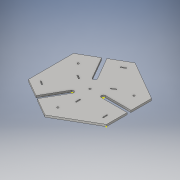
# Autodesk Inventor part: servo mount
Saved by Autodesk Inventor 2016 (Build 200138000, 138)
## iProperties
Created: 2016-04-10
Part Number: servo mount
Material: Generic
Document SubType Name: Modeling
Designer: Sam
Density: 1 g/cm^3
Appearance: Default
Author: Sam
Autodesk Inventor part; units mm, degrees
ref_plane "YZ Plane" through (0, 0, 0) normal (1, 0, 0) x (0, 1, 0)
ref_plane "XZ Plane" through (0, 0, 0) normal (0, 1, 0) x (-1, 0, 0)
ref_plane "XY Plane" through (0, 0, 0) normal (0, 0, 1) x (1, 0, 0)
sketch "Sketch1" plane through (0, 0, 0) normal (0, 1, 0) x (-1, 0, 0)
  point P0 (0, 0)
sketch "Sketch2" plane through (0, 0, 0) normal (0, 1, 0) x (-1, 0, 0)
  line L0 (0, 0) -> (0, -70)
  line L1 (0, -70) -> (54.3409, -70) construction
  line L2 (0, -70) -> (60.6218, -105)
  line L3 (0, -70) -> (70, -70) construction
  line L4 (60.6218, -105) -> (121.2436, -70)
  line L5 (121.2436, -70) -> (121.2436, 0)
  line L6 (121.2436, 0) -> (60.6218, 35)
  line L7 (60.6218, 35) -> (0, 0)
  dimension "d0" = 70
  dimension "d2" = 70
  dimension "d3" = 30
  dimension "d4" = 70
  dimension "d5" = 120
  dimension "d6" = 70
  dimension "d7" = 120
  constraints: 16 end point, 2 horizontal, 2 parallel, 2 vertical, 1 equal length
  measures "d0" distance of L0.start L0.end
  measures "d2" distance of L0.end L2.end
  measures "d3" angle of L2 L3
  measures "d4" distance of L2.end L4.end
  measures "d5" angle of L4 L2
  measures "d6" distance of L5.end L6.end
  measures "d7" angle of L6 L5
extrude "Extrusion1" add sketch "Sketch2" along normal blind 3
sketch "Sketch3" plane through (0, 3, 0) normal (0, 1, 0) x (1, 0, 0)
  line L0 (0, 0) -> (0, 70) projected
  line L1 (-121.2436, 0) -> (-60.6218, -35) projected
  line L2 (-90.9327, -17.5) -> (-50.9327, -17.5) construction
  line L3 (-60.6218, 105) -> (-121.2436, 70) projected
  line L4 (-90.9327, 87.5) -> (-50.9327, 87.5) construction
  line L5 (-70.9327, 17.141) -> (-90.9327, -17.5) construction
  line L6 (-73.5307, 18.641) -> (-93.5307, -16)
  line L7 (-88.3346, -19) -> (-68.3346, 15.641)
  arc A0 (-68.3346, 15.641) -> (-73.5307, 18.641) centre (-70.9327, 17.141) ccw
  arc A1 (-93.5307, -16) -> (-88.3346, -19) centre (-90.9327, -17.5) ccw
  line L8 (-70.9327, 52.859) -> (-90.9327, 87.5) construction
  line L9 (-68.3346, 54.359) -> (-88.3346, 89)
  line L10 (-93.5307, 86) -> (-73.5307, 51.359)
  arc A2 (-73.5307, 51.359) -> (-68.3346, 54.359) centre (-70.9327, 52.859) ccw
  arc A3 (-88.3346, 89) -> (-93.5307, 86) centre (-90.9327, 87.5) ccw
  line L11 (-40, 35) -> (0, 35) construction
  line L12 (-40, 32) -> (0, 32)
  line L13 (0, 38) -> (-40, 38)
  arc A4 (-40, 38) -> (-40, 32) centre (-40, 35) ccw
  arc A5 (0, 32) -> (0, 38) centre (0, 35) ccw
  point P0 (-80.9327, -0.1795)
  point P1 (-80.9327, 70.1795)
  point P2 (-20, 35)
  dimension "d10" = 40
  dimension "d11" = 40
  dimension "d13" = 40
  dimension "d15" = 6
  dimension "d16" = 6
  dimension "d17" = 6
  constraints: 28 end point, 12 point on circle, 12 tangent, 6 centre point, 6 midpoint, 3 parallel, 2 horizontal, 1 perpendicular
  measures "d10" distance of L11.end L11.start
  measures "d11" distance of L2.start L5.start
  measures "d13" distance of L4.start L8.start
  measures "d15" diameter of A1
  measures "d16" diameter of A3
  measures "d17" diameter of A5
extrude "Extrusion3" cut sketch "Sketch3" against normal blind 3
sketch "Sketch4" plane through (0, 3, 0) normal (0, 1, 0) x (1, 0, 0)
  line L0 (-54, 7) -> (-54, 13) construction
  line L1 (-53.25, 7) -> (-53.25, 13)
  line L2 (-54.75, 13) -> (-54.75, 7)
  arc A0 (-54.75, 7) -> (-53.25, 7) centre (-54, 7) ccw
  arc A1 (-53.25, 13) -> (-54.75, 13) centre (-54, 13) ccw
  line L3 (-54, 10) -> (-48, 10) construction
  line L4 (-12, 7) -> (-12, 13) construction
  line L5 (-11.25, 7) -> (-11.25, 13)
  line L6 (-12.75, 13) -> (-12.75, 7)
  arc A2 (-12.75, 7) -> (-11.25, 7) centre (-12, 7) ccw
  arc A3 (-11.25, 13) -> (-12.75, 13) centre (-12, 13) ccw
  line L7 (-12, 10) -> (-6, 10) construction
  arc A4 (-40, 38) -> (-40, 32) centre (-40, 35) ccw projected
  line L8 (-121.2436, 70) -> (-121.2436, 0) projected
  arc A5 (-73.5307, 51.359) -> (-68.3346, 54.359) centre (-70.9327, 52.859) ccw projected
  line L9 (-60.6218, -35) -> (0, 0) projected
  line L10 (-42.282, 53.2346) -> (-45.282, 58.4308) construction
  line L11 (-39.684, 54.7346) -> (-44.8801, 51.7346) construction
  arc A6 (-45.2551, 52.3841) -> (-44.5051, 51.0851) centre (-44.8801, 51.7346) ccw
  line L12 (-44.5051, 51.0851) -> (-39.309, 54.0851)
  arc A7 (-39.309, 54.0851) -> (-40.059, 55.3841) centre (-39.684, 54.7346) ccw
  line L13 (-40.059, 55.3841) -> (-45.2551, 52.3841)
  line L14 (-65.5051, 87.4582) -> (-60.309, 90.4582)
  arc A8 (-60.309, 90.4582) -> (-61.059, 91.7572) centre (-60.684, 91.1077) ccw
  arc A9 (-66.2551, 88.7572) -> (-65.5051, 87.4582) centre (-65.8801, 88.1077) ccw
  line L15 (-60.684, 91.1077) -> (-65.8801, 88.1077) construction
  line L16 (-61.059, 91.7572) -> (-66.2551, 88.7572)
  line L17 (-63.282, 89.6077) -> (-66.282, 94.8038) construction
  line L18 (-85.5833, 41.7654) -> (-88.5833, 36.5692) construction
  line L19 (-88.1814, 43.2654) -> (-82.9852, 40.2654) construction
  arc A10 (-83.3602, 39.6159) -> (-82.6102, 40.9149) centre (-82.9852, 40.2654) ccw
  line L20 (-82.6102, 40.9149) -> (-87.8064, 43.9149)
  arc A11 (-87.8064, 43.9149) -> (-88.5564, 42.6159) centre (-88.1814, 43.2654) ccw
  line L21 (-88.5564, 42.6159) -> (-83.3602, 39.6159)
  line L22 (-103.6102, 4.5418) -> (-108.8064, 7.5418)
  arc A12 (-108.8064, 7.5418) -> (-109.5564, 6.2428) centre (-109.1814, 6.8923) ccw
  arc A13 (-104.3602, 3.2428) -> (-103.6102, 4.5418) centre (-103.9852, 3.8923) ccw
  line L23 (-109.1814, 6.8923) -> (-103.9852, 3.8923) construction
  line L24 (-109.5564, 6.2428) -> (-104.3602, 3.2428)
  line L25 (-106.5833, 5.3923) -> (-109.5833, 0.1962) construction
  point P0 (-60.6218, 35)
  dimension "d25" = 3
  dimension "d27" = 1.5
  dimension "d29" = 3
  dimension "d31" = 1.5
  dimension "d48" = 360
  constraints: 60 end point, 24 point on circle, 12 centre point, 8 tangent, 2 horizontal, 2 midpoint, 2 parallel, 2 perpendicular, 85 other
  measures "d25" distance of L3.start L0.end
  measures "d27" diameter of A1
  measures "d29" distance of L7.start L4.end
  measures "d31" diameter of A3
extrude "Extrusion4" cut sketch "Sketch4" against normal blind 10
sketch "Sketch5" plane through (0, 0, 0) normal (0, -1, 0) x (1, 0, 0)
  arc A0 (-73.5307, -18.641) -> (-68.3346, -15.641) centre (-70.9327, -17.141) ccw projected
  line L0 (-70.9327, -17.141) -> (-50.3109, -17.141) construction
  arc A1 (-40, -32) -> (-40, -38) centre (-40, -35) ccw projected
  point P0 (0, 0)
  point P1 (-60.6218, -35)
  constraints: 2 end point, 1 horizontal
sketch "Sketch6" plane through (0, 3, 0) normal (0, 1, 0) x (1, 0, 0)
  line L0 (-60.6218, -35) -> (0, 0) projected
  circle A0 centre (-60.6218, -15) radius 1.4
  circle A1 centre (-17.3205, 60) radius 1.4
  circle A2 centre (-103.923, 60) radius 1.4
  circle A3 centre (-60.6218, 35) radius 1.4
  dimension "d52" = 2.8
  dimension "d55" = 360
  dimension "d57" = 2.8
  constraints: 4 centre point, 1 coincident, 7 other
  measures "d52" diameter of A0
  measures "d57" diameter of A3
extrude "Extrusion5" cut sketch "Sketch6" against normal blind 10
body "Solid1"
